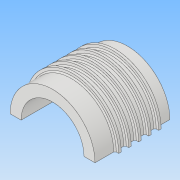
# Autodesk Inventor part: CoreOpposite
Saved by Autodesk Inventor 2017.3 (Build 213256000, 256)
## iProperties
Created: 2019-06-19
Part Number: CoreOpposite
Material: ABS Plastic
Document SubType Name: Modeling
Designer: Derek Wider
Density: 1.06 g/cm^3
Appearance: Smooth - White
Author: Derek Wider
Autodesk Inventor part; units mm, degrees
ref_plane "YZ Plane" through (0, 0, 0) normal (1, 0, 0) x (0, 1, 0)
ref_plane "XZ Plane" through (0, 0, 0) normal (0, 1, 0) x (-1, 0, 0)
ref_plane "XY Plane" through (0, 0, 0) normal (0, 0, 1) x (1, 0, 0)
sketch "Sketch1" plane through (0, 0, 0) normal (0, 0, 1) x (1, 0, 0)
  arc A0 (16.002, 0) -> (-16.002, 0) centre (0, 0) ccw
  arc A1 (21.59, 0) -> (-21.59, 0) centre (0, 0) ccw
  line L0 (-16.002, 0) -> (-21.59, 0)
  line L1 (16.002, 0) -> (21.59, 0)
  dimension "d0" = 43.18
  dimension "d1" = 32.004
  constraints: 4 end point, 4 point on circle, 2 centre point, 2 coincident, 2 point on line, 1 horizontal
  measures "d0" diameter of A1
  measures "d1" diameter of A0
extrude "Extrusion1" add sketch "Sketch1" along normal blind 38.1
ref_plane "Work Plane1" through (0, 0, 27.94) normal (0, 0, 1) x (1, 0, 0)
sketch "Sketch2" plane through (0, 0, 27.94) normal (0, 0, 1) x (1, 0, 0)
  arc A0 (21.59, 0) -> (-21.59, 0) centre (0, 0) ccw projected
  arc A1 (23.495, 0) -> (-23.495, 0) centre (0, 0) ccw
  line L0 (-21.59, 0) -> (-23.495, 0)
  line L1 (16.002, 0) -> (21.59, 0) projected
  line L2 (23.495, 0) -> (21.59, 0)
  dimension "d5" = 1.905
  constraints: 4 end point, 2 point on circle, 1 centre point, 1 collinear
  measures "d5" distance of L0.end L0.start
extrude "Extrusion2" add sketch "Sketch2" against normal blind 1.27
chamfer "Chamfer1" distance 0.635 angle 45 2 edges at (0, 21.59, 27.94) (0, 21.59, 26.67)
pattern_linear "Rectangular Pattern1" count 5 spacing 5.08 along (0, 0, -1) of "Extrusion2", "Chamfer1"
body "Solid1"
